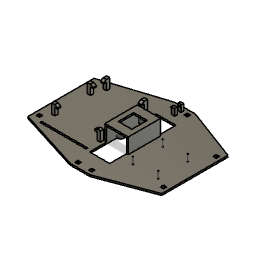
Seismo-Case v4 (Autodesk Fusion 360 design; units mm, degrees)
Autodesk Fusion 360 part; units mm, degrees
note: some values were not read from the file. Set by a fixed rule: which sketch regions a step uses.
sketch "Sketch1" plane through (0, 0, 0) normal (0, 1, 0) x (1, 0, 0)
  line L0 (-20, 30) -> (25.5, 30)
  line L1 (25.5, 30) -> (25.5, -33)
  line L2 (25.5, -33) -> (-20, -33)
  line L3 (-20, -33) -> (-20, 30)
  dimension "d1" = 63
  dimension "d2" = 45.5
  constraint horizontal L0
  constraint vertical L1
  constraint horizontal L2
  constraint vertical L3
  measures "d1" distance of L0.start L2.end
  measures "d2" distance of L0.start L0.end
extrude "Extrude1" add sketch "Sketch1" along normal blind 3.175 makes body 1
sketch "Sketch2" plane through (0, 0, 0) normal (0, -1, 0) x (1, 0, 0)
  line L0 (25.5, 33) -> (-20, 33)
  line L1 (-20, 33) -> (-20, -30)
  line L2 (-20, -30) -> (25.5, -30)
  line L3 (25.5, -30) -> (25.5, 33)
  circle A0 centre (2.225, 23.875) radius 6.2
  circle A1 centre (2.225, -20.875) radius 6.2
  dimension "d5" = 12.4
  dimension "d6" = 9.125
  dimension "d7" = 22.225
  dimension "d8" = 12.4
  dimension "d9" = 9.125
  dimension "d10" = 22.225
  measures "d5" diameter of A0
  measures "d6" distance of L0 A0.centre
  measures "d7" distance of L1 A0.centre
  measures "d8" diameter of A1
  measures "d9" distance of L2 A1.centre
  measures "d10" distance of L1 A1.centre
extrude "Extrude2" add sketch "Sketch2" along normal blind 12.065 contours A0 | A1 bodies 1
sketch "Sketch3" plane through (0, 0, 0) normal (0, -1, 0) x (1, 0, 0)
  circle A0 centre (2.225, -20.875) radius 6.2
  circle A1 centre (2.225, 23.875) radius 6.2
  line L0 (25.5, 33) -> (-20, 33)
  line L1 (-20, 33) -> (-20, -30)
  line L2 (-20, -30) -> (25.5, -30)
  line L3 (25.5, -30) -> (25.5, 33)
  line L4 (25.5, 33) -> (22.325, 33)
  line L5 (22.325, 33) -> (22.325, -30)
  line L6 (22.325, -30) -> (25.5, -30)
  line L7 (25.5, -30) -> (25.5, 33)
  line L8 (-20, 33) -> (-16.825, 33)
  line L9 (-16.825, 33) -> (-16.825, -30)
  line L10 (-16.825, -30) -> (-20, -30)
  line L11 (-20, -30) -> (-20, 33)
  dimension "d13" = 3.175
  dimension "d14" = 3.175
  constraint horizontal L4
  constraint vertical L5
  constraint horizontal L6
  constraint vertical L7
  constraint coincident L2 L5.end
  constraint coincident L0.start L3.end
  constraint horizontal L8
  constraint vertical L9
  constraint horizontal L10
  constraint vertical L11
  constraint coincident L0.end L1.start
  measures "d13" distance of L5 L7
  measures "d14" distance of L0.end L8.end
extrude "Extrude3" add sketch "Sketch3" along normal blind 26.67 contours L0 L2 L3 L4 L5 L6 L7 | L0 L1 L2 L8 L9 L10 L11 bodies 1
sketch "Sketch4" plane through (0, 3.175, 0) normal (0, 1, 0) x (-1, 0, 0)
  line L0 (20, 33) -> (-25.5, 33)
  line L1 (-25.5, 33) -> (-25.5, -30)
  line L2 (-25.5, -30) -> (20, -30)
  line L3 (20, -30) -> (20, 33)
  line L4 (10.475, -13.5) -> (-15.975, -13.5)
  line L5 (-15.975, -13.5) -> (-15.975, 16.5)
  line L6 (-15.975, 16.5) -> (10.475, 16.5)
  line L7 (10.475, 16.5) -> (10.475, -13.5)
  dimension "d17" = 16.5
  dimension "d18" = 16.5
  dimension "d19" = 9.525
  dimension "d20" = 9.525
  constraint horizontal L4
  constraint vertical L5
  constraint horizontal L6
  constraint vertical L7
  measures "d17" distance of L2 L4
  measures "d18" distance of L0 L6
  measures "d19" distance of L3 L7
  measures "d20" distance of L1 L5
extrude "Extrude4" cut sketch "Sketch4" against normal blind 22 contours L4 L5 L6 L7 bodies 1
ref_plane "WorkPlane1" through (23.9125, -26.67, 1.5) normal (0, -1, 0) x (0, 0, -1)
sketch "Sketch5" plane through (23.9125, -26.67, 1.5) normal (0, -1, 0) x (1, 0, 0)
  line L0 (-1.5875, -31.5) -> (-1.5875, -64.5)
  line L1 (-1.5875, 31.6383) -> (-1.5875, 64.6383)
  line L2 (-40.7375, 31.6383) -> (-40.7375, 64.6383)
  line L3 (-40.7375, -31.5) -> (-40.7375, -64.5)
  line L4 (-40.7375, -64.5) -> (-1.5875, -64.5)
  line L5 (-1.5875, 64.6383) -> (-40.7375, 64.6383)
  line L6 (-1.5875, -102.6) -> (100.0125, -64.5)
  line L7 (-1.5875, 102.7383) -> (100.0125, 64.6383)
  line L8 (-1.5875, -102.6) -> (-40.7375, -102.6)
  line L9 (-1.5875, 102.7383) -> (-40.7375, 102.7383)
  line L10 (-40.7375, 102.7383) -> (-160.7372, 64.9242)
  line L11 (100.0125, 64.6383) -> (100.0125, -64.5)
  line L12 (-1.5875, 31.6383) -> (-1.5875, 31.5)
  line L13 (-1.5875, 31.5) -> (1.6, 31.5)
  line L14 (1.6, 31.5) -> (1.6, -31.5)
  line L15 (-43.9125, -31.5) -> (-43.9125, 31.5)
  line L16 (-40.7375, 31.6383) -> (-40.7375, 31.5)
  line L17 (-40.7375, 31.5) -> (-43.9125, 31.5)
  line L18 (1.6, -31.5) -> (-1.5875, -31.5)
  line L19 (-40.7375, -31.5) -> (-43.9125, -31.5)
  line L20 (-160.7372, 64.9242) -> (-160.7372, -64.2138)
  line L21 (-40.7375, -102.6) -> (-160.7372, -64.2138)
  point P0 (-1.5875, -31.5)
  point P1 (-1.5875, 31.6383)
  point P2 (-43.9125, -31.5)
  point P3 (-43.9125, 31.5)
  point P4 (-40.7375, -31.5)
  point P5 (-40.7375, 31.6383)
  dimension "d28" = 33
  dimension "d29" = 33
  dimension "d30" = 33
  dimension "d31" = 33
  dimension "d32" = 38.1
  dimension "d35" = 101.6
  dimension "d37" = 38.1
  dimension "d38" = 120
  dimension "d40" = 38.1
  dimension "d41" = 38.1
  dimension "d42" = 129.1383
  dimension "d68" = 129.138
  constraint coincident P0 L0.start
  constraint coincident P1 L1.start
  constraint coincident P5 L2.start
  constraint vertical L2
  constraint coincident P4 L3.start
  constraint vertical L3
  constraint perpendicular L0 L4
  constraint perpendicular L1 L5
  constraint parallel L1 L12
  constraint perpendicular L13 L14
  constraint coincident P2 L15.start
  constraint coincident P3 L15.end
  constraint parallel L3 L15
  constraint parallel L15 L16
  constraint perpendicular L15 L17
  constraint perpendicular L15 L19
  constraint vertical L20
  measures "d28" distance of P0 L0.end
  measures "d29" distance of P1 L1.end
  measures "d30" distance of P5 L2.end
  measures "d31" distance of P4 L3.end
  measures "d32" distance of L0.end L6.start
  measures "d35" distance of L0.end L6.end
  measures "d37" distance of L1.end L7.start
  measures "d38" distance of L2.end L10.end
  measures "d40" distance of L3.end L8.end
  measures "d41" distance of L2.end L9.end
  measures "d42" distance of L6.end L7.end
  measures "d68" distance of L10.end L20.end
extrude "Extrude5" add sketch "Sketch5" along normal blind 3.175 separate body makes body 2
sketch "Sketch6" plane through (0, -26.67, 0) normal (0, 1, 0) x (-1, 0, 0)
  line L0 (16.825, -63) -> (-22.325, -63)
  line L1 (-22.325, -63) -> (-22.325, -30)
  line L2 (-22.325, -30) -> (-25.5125, -30)
  line L3 (-25.5125, -30) -> (-25.5125, 33)
  line L4 (-25.5125, 33) -> (-22.325, 33)
  line L5 (-22.325, 33) -> (-22.325, 66.1383)
  line L6 (-22.325, 66.1383) -> (16.825, 66.1383)
  line L7 (16.825, 66.1383) -> (16.825, 33)
  line L8 (16.825, 33) -> (20, 33)
  line L9 (20, 33) -> (20, -30)
  line L10 (20, -30) -> (16.825, -30)
  line L11 (16.825, -30) -> (16.825, -63)
  line L12 (16.825, 104.2383) -> (-22.325, 104.2383)
  line L13 (-22.325, 104.2383) -> (-123.925, 66.1383)
  line L14 (-123.925, 66.1383) -> (-123.925, -63)
  line L15 (-123.925, -63) -> (-22.325, -101.1)
  line L16 (-22.325, -101.1) -> (16.825, -101.1)
  line L17 (136.8247, 66.4242) -> (16.825, 104.2383)
  line L18 (0.425, -95) -> (-5.925, -95)
  line L19 (-5.925, -95) -> (-5.925, -89.92)
  line L20 (-5.925, -89.92) -> (0.425, -89.92)
  line L21 (0.425, -89.92) -> (0.425, -95)
  line L22 (0.425, -82.3) -> (-5.925, -82.3)
  line L23 (-5.925, -82.3) -> (-5.925, -77.22)
  line L24 (-5.925, -77.22) -> (0.425, -77.22)
  line L25 (0.425, -77.22) -> (0.425, -82.3)
  line L26 (16.825, -101.1) -> (136.8247, -62.7138)
  line L27 (136.8247, -62.7138) -> (136.8247, 66.4242)
  dimension "d45" = 6.35
  dimension "d46" = 5.08
  dimension "d48" = 16.4
  dimension "d50" = 6.35
  dimension "d51" = 5.08
  dimension "d52" = 16.4
  dimension "d53" = 7.62
  constraint horizontal L18
  constraint vertical L19
  constraint horizontal L20
  constraint vertical L21
  constraint horizontal L22
  constraint vertical L23
  constraint horizontal L24
  constraint vertical L25
  measures "d45" distance of L18.start L18.end
  measures "d46" distance of L18.end L19.end
  measures "d48" distance of L11 L21
  measures "d50" distance of L22.start L22.end
  measures "d51" distance of L22.end L23.end
  measures "d52" distance of L11 L25
  measures "d53" distance of L20 L22
extrude "Extrude6" add sketch "Sketch6" along normal blind 12.7 contours L18 L19 L20 L21 | L22 L23 L24 L25 bodies 2
sketch "Sketch7" plane through (5.925, 0, 0) normal (1, 0, 0) x (0, 0, -1)
  line L0 (77.22, -26.67) -> (82.3, -26.67)
  line L1 (82.3, -26.67) -> (82.3, -13.97)
  line L2 (82.3, -13.97) -> (77.22, -13.97)
  line L3 (77.22, -13.97) -> (77.22, -26.67)
  line L4 (83.57, -16) -> (83.57, -17)
  line L5 (88.65, -16) -> (88.65, -17)
  line L6 (83.57, -16) -> (82.3, -13.97)
  line L7 (83.57, -17) -> (82.3, -17)
  line L8 (88.65, -17) -> (89.92, -17)
  line L9 (89.92, -13.97) -> (88.65, -16)
  line L10 (89.92, -13.97) -> (89.92, -17)
  point P0 (89.92, -13.97)
  dimension "d56" = 5.08
  dimension "d58" = 1.27
  constraint perpendicular L2 L4
  constraint vertical L5
  constraint coincident L1.end L2.start
  constraint coincident L1 L7.end
  constraint perpendicular L1 L7
  constraint perpendicular L5 L8
  constraint coincident P0 L9.start
  constraint perpendicular L8 L10
  measures "d56" distance of L4.start L5.start
  measures "d58" distance of L1 L4.start
extrude "Extrude7" add sketch "Sketch7" against normal blind 6.35 contours L1 L4 L6 L7 | L5 L8 L9 L10 bodies 2
sketch "Sketch8" plane through (0, -26.67, 0) normal (0, 1, 0) x (-1, 0, 0)
  line L0 (0.425, -77.22) -> (0.425, -82.3)
  line L1 (0.425, -82.3) -> (-5.925, -82.3)
  line L2 (-5.925, -82.3) -> (-5.925, -77.22)
  line L3 (-5.925, -77.22) -> (0.425, -77.22)
  line L4 (0.425, -89.92) -> (0.425, -95)
  line L5 (0.425, -95) -> (-5.925, -95)
  line L6 (-5.925, -95) -> (-5.925, -89.92)
  line L7 (-5.925, -89.92) -> (0.425, -89.92)
  line L8 (16.825, -63) -> (-22.325, -63)
  line L9 (-22.325, -63) -> (-22.325, -30)
  line L10 (-22.325, -30) -> (-25.5125, -30)
  line L11 (-25.5125, -30) -> (-25.5125, 33)
  line L12 (-25.5125, 33) -> (-22.325, 33)
  line L13 (-22.325, 33) -> (-22.325, 66.1383)
  line L14 (-22.325, 66.1383) -> (16.825, 66.1383)
  line L15 (16.825, 66.1383) -> (16.825, 33)
  line L16 (16.825, 33) -> (20, 33)
  line L17 (20, 33) -> (20, -30)
  line L18 (20, -30) -> (16.825, -30)
  line L19 (16.825, -30) -> (16.825, -63)
  line L20 (16.825, 104.2383) -> (-22.325, 104.2383)
  line L21 (-22.325, 104.2383) -> (-123.925, 66.1383)
  line L22 (-123.925, 66.1383) -> (-123.925, -63)
  line L23 (-123.925, -63) -> (-22.325, -101.1)
  line L24 (-22.325, -101.1) -> (16.825, -101.1)
  line L25 (136.8247, 66.4242) -> (16.825, 104.2383)
  line L26 (111.4247, -51.1) -> (28.8747, -51.1)
  line L27 (28.8747, -51.1) -> (28.8747, 65.105)
  line L28 (28.8747, 65.105) -> (111.4247, 65.105)
  line L29 (111.4247, 65.105) -> (111.4247, -51.1)
  line L30 (16.825, -101.1) -> (136.8247, -62.7138)
  line L31 (136.8247, -62.7138) -> (136.8247, 66.4242)
  line L32 (59.9342, -51.1) -> (59.9342, -70.15)
  line L33 (114.5997, 68.28) -> (25.6997, 68.28)
  line L34 (25.6997, 68.28) -> (25.6997, 65.105)
  line L35 (25.6997, 65.105) -> (28.8747, 65.105)
  line L36 (114.5997, 68.28) -> (114.5997, 65.105)
  line L37 (114.5997, 65.105) -> (111.4247, 65.105)
  line L38 (-34.3875, -41.7617) -> (-94.3875, -41.7617)
  line L39 (-94.3875, -41.7617) -> (-94.3875, 47.2383)
  line L40 (-94.3875, 47.2383) -> (-34.3875, 47.2383)
  line L41 (-34.3875, 47.2383) -> (-34.3875, -41.7617)
  line L42 (28.8747, 33) -> (22.5247, 33)
  line L43 (22.5247, 33) -> (22.5247, 39.35)
  line L44 (22.5247, 39.35) -> (28.8747, 39.35)
  line L45 (28.8747, 39.35) -> (28.8747, 33)
  line L46 (111.4247, 33) -> (117.7747, 33)
  line L47 (117.7747, 33) -> (117.7747, 39.35)
  line L48 (117.7747, 39.35) -> (111.4247, 39.35)
  line L49 (111.4247, 39.35) -> (111.4247, 33)
  line L50 (28.8747, -30.0326) -> (22.5247, -30.0326)
  line L51 (22.5247, -30.0326) -> (22.5247, -36.3826)
  line L52 (22.5247, -36.3826) -> (28.8747, -36.3826)
  line L53 (28.8747, -36.3826) -> (28.8747, -30.0326)
  line L54 (111.4247, -36.3826) -> (117.7747, -36.3826)
  line L55 (117.7747, -36.3826) -> (117.7747, -30.0326)
  line L56 (117.7747, -30.0326) -> (111.4247, -30.0326)
  line L57 (111.4247, -30.0326) -> (111.4247, -36.3826)
  dimension "d61" = 82.55
  dimension "d62" = 116.205
  dimension "d64" = 50
  dimension "d65" = 39.1333
  dimension "d69" = 25.4
  dimension "d70" = 19.05
  dimension "d71" = 3.175
  dimension "d72" = 3.175
  dimension "d73" = 3.175
  dimension "d74" = 89
  dimension "d75" = 60
  dimension "d78" = 57
  dimension "d79" = 59.3383
  dimension "d80" = 6.35
  dimension "d81" = 6.35
  dimension "d82" = 8.8747
  dimension "d83" = 8.875
  dimension "d84" = 6.35
  dimension "d85" = 6.35
  dimension "d86" = 6.35
  dimension "d87" = 6.35
  dimension "d88" = 6.35
  dimension "d89" = 6.35
  constraint horizontal L26
  constraint vertical L27
  constraint horizontal L28
  constraint vertical L29
  constraint coincident L26 L32.start
  constraint perpendicular L26 L32
  constraint perpendicular L29 L33
  constraint perpendicular L33 L34
  constraint perpendicular L27 L35
  constraint perpendicular L33 L36
  constraint perpendicular L36 L37
  constraint horizontal L38
  constraint vertical L39
  constraint horizontal L40
  constraint vertical L41
  constraint horizontal L42
  constraint vertical L43
  constraint horizontal L44
  constraint vertical L45
  constraint coincident L27 L42.start
  constraint horizontal L46
  constraint vertical L47
  constraint horizontal L48
  constraint vertical L49
  constraint coincident L29 L46.start
  constraint horizontal L50
  constraint vertical L51
  constraint horizontal L52
  constraint vertical L53
  constraint coincident L27 L50.start
  constraint horizontal L54
  constraint vertical L55
  constraint horizontal L56
  constraint vertical L57
  constraint coincident L29 L54.start
  measures "d61" distance of L26.start L26.end
  measures "d62" distance of L26.start L28.end
  measures "d64" distance of L24 L26
  measures "d65" distance of L20 L28
  measures "d69" distance of L29 L31
  measures "d70" distance of L32.start L32.end
  measures "d71" distance of L28 L33
  measures "d72" distance of L29 L36
  measures "d73" distance of L27 L34
  measures "d74" distance of L38.end L39.end
  measures "d75" distance of L39.end L40.end
  measures "d78" distance of L20 L40
  measures "d79" distance of L24 L38
  measures "d80" distance of L42.start L42.end
  measures "d81" distance of L42 L44
  measures "d82" distance of L17 L27
  measures "d83" distance of L11 L41
  measures "d84" distance of L46.start L46.end
  measures "d85" distance of L46 L48
  measures "d86" distance of L50.start L50.end
  measures "d87" distance of L50 L52
  measures "d88" distance of L54.start L54.end
  measures "d89" distance of L54 L56
extrude "Extrude8" add sketch "Sketch8" along normal blind 19.05 contours L29 L54 L55 L56 L57 | L27 L50 L51 L52 L53 | L29 L46 L47 L48 L49 | L27 L42 L43 L44 L45 bodies 2
sketch "Sketch9" plane through (0, 0, 39.35) normal (0, 0, 1) x (1, 0, 0)
  line L0 (-117.7747, -26.67) -> (-111.4247, -26.67)
  line L1 (-111.4247, -26.67) -> (-111.4247, -7.62)
  line L2 (-111.4247, -7.62) -> (-117.7747, -7.62)
  line L3 (-117.7747, -7.62) -> (-117.7747, -26.67)
  line L4 (-111.4247, -7.62) -> (-105.9254, -10.795)
  line L5 (-105.9254, -10.795) -> (-105.9254, -12.3825)
  line L6 (-105.9254, -12.3825) -> (-111.4247, -12.3825)
  line L7 (-111.4247, -7.62) -> (-111.4247, -12.3825)
  line L8 (-34.3739, -10.795) -> (-34.3739, -12.383)
  line L9 (-28.8747, -7.62) -> (-34.3739, -10.795)
  line L10 (-28.8747, -7.62) -> (-28.8747, -12.383)
  line L11 (-28.8747, -12.383) -> (-34.3739, -12.383)
  point P0 (-28.8747, -7.62)
  dimension "d92" = 6.35
  dimension "d93" = 120
  dimension "d94" = 1.5875
  dimension "d98" = 1.588
  dimension "d101" = 6.35
  dimension "d102" = 90
  dimension "d103" = 120
  constraint coincident L1.end L2.start
  constraint vertical L5
  constraint coincident L1 L6.end
  constraint perpendicular L1 L6
  constraint vertical L8
  constraint coincident P0 L9.start
  constraint vertical L10
  measures "d92" distance of L1.end L4.end
  measures "d93" angle of L1 L4
  measures "d94" distance of L4.end L5.end
  measures "d98" distance of L8.start L8.end
  measures "d101" distance of L8.start P0
  measures "d102" angle of L10 L11
  measures "d103" angle of L9 L10
extrude "Extrude9" add sketch "Sketch9" against normal blind 6.35 contours L1 L4 L5 L6 L7 | L8 L9 L10 L11 bodies 2
sketch "Sketch10" plane through (0, 0, -36.3826) normal (0, 0, -1) x (-1, 0, 0)
  line L0 (22.5247, -26.67) -> (28.8747, -26.67)
  line L1 (28.8747, -26.67) -> (28.8747, -7.62)
  line L2 (28.8747, -7.62) -> (22.5247, -7.62)
  line L3 (22.5247, -7.62) -> (22.5247, -26.67)
  line L4 (28.8747, -7.62) -> (34.3739, -10.795)
  line L5 (34.3739, -10.795) -> (34.3739, -12.3825)
  line L6 (34.3739, -12.3825) -> (28.8747, -12.3825)
  line L7 (28.8747, -7.62) -> (28.8747, -12.3825)
  dimension "d107" = 6.35
  dimension "d108" = 120
  dimension "d109" = 1.5875
  constraint coincident L1.end L2.start
  constraint parallel L1 L5
  constraint coincident L1 L6.end
  constraint perpendicular L1 L6
  constraint perpendicular L6 L7
  measures "d107" distance of L1.end L4.end
  measures "d108" angle of L4 L7
  measures "d109" distance of L4.end L5.end
extrude "Extrude10" add sketch "Sketch10" against normal blind 6.35 contours L1 L4 L5 L6 L7 bodies 2
sketch "Sketch11" plane through (0, 0, -30.0326) normal (0, 0, 1) x (1, 0, 0)
  line L0 (-117.7747, -26.67) -> (-111.4247, -26.67)
  line L1 (-111.4247, -26.67) -> (-111.4247, -7.62)
  line L2 (-111.4247, -7.62) -> (-117.7747, -7.62)
  line L3 (-117.7747, -7.62) -> (-117.7747, -26.67)
  line L4 (-111.4247, -7.62) -> (-105.9212, -10.7878)
  line L5 (-105.9212, -10.7878) -> (-105.9212, -12.4)
  line L6 (-105.9212, -12.4) -> (-111.4247, -12.4)
  line L7 (-111.4247, -7.62) -> (-111.4247, -12.4)
  dimension "d113" = 6.35
  constraint coincident L1.end L2.start
  constraint vertical L5
  constraint coincident L1 L6.end
  constraint perpendicular L1 L6
  measures "d113" distance of L1.end L4.end
extrude "Extrude11" add sketch "Sketch11" against normal blind 6.35 contours L1 L4 L5 L6 L7 bodies 2
sketch "Sketch12" plane through (0, -29.845, 0) normal (0, -1, 0) x (1, 0, 0)
  line L0 (22.325, -63) -> (-16.825, -63)
  line L1 (-16.825, -63) -> (-16.825, -30)
  line L2 (-16.825, -30) -> (-20, -30)
  line L3 (-20, -30) -> (-20, 33)
  line L4 (-20, 33) -> (-16.825, 33)
  line L5 (-16.825, 33) -> (-16.825, 66.1383)
  line L6 (-16.825, 66.1383) -> (22.325, 66.1383)
  line L7 (22.325, 66.1383) -> (22.325, 33)
  line L8 (22.325, 33) -> (25.5125, 33)
  line L9 (25.5125, 33) -> (25.5125, -30)
  line L10 (25.5125, -30) -> (22.325, -30)
  line L11 (22.325, -30) -> (22.325, -63)
  line L12 (22.325, -101.1) -> (123.925, -63)
  line L13 (123.925, -63) -> (123.925, 66.1383)
  line L14 (123.925, 66.1383) -> (22.325, 104.2383)
  line L15 (22.325, 104.2383) -> (-16.825, 104.2383)
  line L16 (-16.825, 104.2383) -> (-136.8247, 66.4242)
  line L17 (-136.8247, 66.4242) -> (-136.8247, -62.7138)
  line L18 (-136.8247, -62.7138) -> (-16.825, -101.1)
  line L19 (-16.825, -101.1) -> (22.325, -101.1)
  line L20 (-16.825, 33) -> (-20, 33)
  line L21 (-20, 33) -> (-20, -30)
  line L22 (-20, -30) -> (-16.825, -30)
  line L23 (-16.825, -30) -> (-16.825, 33)
  line L24 (22.325, 33) -> (25.5125, 33)
  line L25 (25.5125, 33) -> (25.5125, -30)
  line L26 (25.5125, -30) -> (22.325, -30)
  line L27 (22.325, -30) -> (22.325, 33)
  constraint horizontal L20
  constraint vertical L21
  constraint horizontal L22
  constraint vertical L23
  constraint coincident L2.end L3.start
  constraint coincident L4.end L5.start
  constraint horizontal L24
  constraint vertical L25
  constraint horizontal L26
  constraint vertical L27
  constraint coincident L9.end L10.start
  constraint coincident L7.end L8.start
extrude "Extrude12" add sketch "Sketch12" against normal blind 3.175 contours L8 L9 L10 L24 L25 L26 L27 | L2 L3 L4 L20 L21 L22 L23 bodies 1 2
sketch "Sketch13" plane through (0, -26.67, 0) normal (0, 1, 0) x (-1, 0, 0)
  line L0 (111.4247, 39.35) -> (117.7747, 39.35)
  line L1 (117.7747, 39.35) -> (117.7747, 33)
  line L2 (117.7747, 33) -> (111.4247, 33)
  line L3 (111.4247, 33) -> (111.4247, 39.35)
  line L4 (111.4247, -30.0326) -> (117.7747, -30.0326)
  line L5 (117.7747, -30.0326) -> (117.7747, -36.3826)
  line L6 (117.7747, -36.3826) -> (111.4247, -36.3826)
  line L7 (111.4247, -36.3826) -> (111.4247, -30.0326)
  line L8 (28.8747, 39.35) -> (28.8747, 33)
  line L9 (28.8747, 33) -> (22.5247, 33)
  line L10 (22.5247, 33) -> (22.5247, 39.35)
  line L11 (22.5247, 39.35) -> (28.8747, 39.35)
  line L12 (28.8747, -36.3826) -> (22.5247, -36.3826)
  line L13 (22.5247, -36.3826) -> (22.5247, -30.0326)
  line L14 (22.5247, -30.0326) -> (28.8747, -30.0326)
  line L15 (28.8747, -30.0326) -> (28.8747, -36.3826)
  line L16 (0.425, -77.22) -> (0.425, -82.3)
  line L17 (0.425, -82.3) -> (-5.925, -82.3)
  line L18 (-5.925, -82.3) -> (-5.925, -77.22)
  line L19 (-5.925, -77.22) -> (0.425, -77.22)
  line L20 (0.425, -89.92) -> (0.425, -95)
  line L21 (0.425, -95) -> (-5.925, -95)
  line L22 (-5.925, -95) -> (-5.925, -89.92)
  line L23 (-5.925, -89.92) -> (0.425, -89.92)
  line L24 (16.825, -63) -> (-22.325, -63)
  line L25 (-22.325, -63) -> (-22.325, -30)
  line L26 (-22.325, -30) -> (-25.5, -30)
  line L27 (-25.5, -30) -> (-25.5, 33)
  line L28 (-25.5, 33) -> (-22.325, 33)
  line L29 (-22.325, 33) -> (-22.325, -30)
  line L30 (-22.325, -30) -> (-22.325, -30)
  line L31 (-22.325, -30) -> (-22.325, 66.1383)
  line L32 (-22.325, 66.1383) -> (16.825, 66.1383)
  line L33 (16.825, 66.1383) -> (16.825, 33)
  line L34 (16.825, 33) -> (20, 33)
  line L35 (20, 33) -> (20, -30)
  line L36 (20, -30) -> (16.825, -30)
  line L37 (16.825, -30) -> (16.825, -63)
  line L38 (-123.925, -63) -> (-22.325, -101.1)
  line L39 (-22.325, -101.1) -> (16.825, -101.1)
  line L40 (16.825, -101.1) -> (136.8247, -62.7138)
  line L41 (136.8247, -62.7138) -> (136.8247, 66.4242)
  line L42 (136.8247, 66.4242) -> (16.825, 104.2383)
  line L43 (16.825, 104.2383) -> (-22.325, 104.2383)
  line L44 (-22.325, 104.2383) -> (-123.925, 66.1383)
  line L45 (-123.925, 66.1383) -> (-123.925, -63)
  line L46 (110, -60) -> (103.65, -60)
  line L47 (103.65, -60) -> (103.65, -53.65)
  line L48 (103.65, -53.65) -> (110, -53.65)
  line L49 (110, -53.65) -> (110, -60)
  line L50 (30, -60) -> (36.35, -60)
  line L51 (36.35, -60) -> (36.35, -53.65)
  line L52 (36.35, -53.65) -> (30, -53.65)
  line L53 (30, -53.65) -> (30, -60)
  line L54 (111.4247, 64.46) -> (28.0914, 64.46)
  dimension "d118" = 6.35
  dimension "d119" = 6.35
  dimension "d120" = 6.35
  dimension "d121" = 6.35
  dimension "d122" = 118.11
  constraint horizontal L46
  constraint vertical L47
  constraint horizontal L48
  constraint vertical L49
  constraint horizontal L50
  constraint vertical L51
  constraint horizontal L52
  constraint vertical L53
  constraint perpendicular L3 L54
  measures "d118" distance of L46.start L46.end
  measures "d119" distance of L46.start L48.end
  measures "d120" distance of L50.start L50.end
  measures "d121" distance of L50.end L51.end
  measures "d122" distance of L48 L54
extrude "Extrude13" add sketch "Sketch13" along normal blind 19.05 contours L46 L47 L48 L49 | L50 L51 L52 L53 bodies 1
sketch "Sketch14" plane through (-110, 0, 0) normal (-1, 0, 0) x (0, 0, 1)
  line L0 (-60, -26.67) -> (-53.65, -26.67)
  line L1 (-53.65, -26.67) -> (-53.65, -7.62)
  line L2 (-53.65, -7.62) -> (-60, -7.62)
  line L3 (-60, -7.62) -> (-60, -26.67)
  line L4 (-48.15, -10.7937) -> (-48.15, -12.3817)
  line L5 (-48.15, -10.7937) -> (-53.65, -7.62)
  line L6 (-48.15, -12.3817) -> (-53.65, -12.3817)
  dimension "d125" = 1.588
  dimension "d126" = 5.5
  dimension "d127" = 6.35
  constraint vertical L4
  constraint coincident L1.end L2.start
  constraint coincident L1 L6.end
  constraint perpendicular L1 L6
  measures "d125" distance of L4.start L4.end
  measures "d126" distance of L1 L4
  measures "d127" distance of L4.start L1.end
extrude "Extrude14" add sketch "Sketch14" against normal blind 6.35 contours L1 L4 L5 L6 bodies 1
sketch "Sketch15" plane through (-30, 0, 0) normal (1, 0, 0) x (0, 0, -1)
  line L0 (53.65, -26.67) -> (60, -26.67)
  line L1 (60, -26.67) -> (60, -7.62)
  line L2 (60, -7.62) -> (53.65, -7.62)
  line L3 (53.65, -7.62) -> (53.65, -26.67)
  line L4 (48.15, -12.3946) -> (48.15, -10.8066)
  line L5 (48.15, -12.3946) -> (53.65, -12.3946)
  line L6 (53.65, -7.62) -> (53.65, -12.3946)
  line L7 (53.65, -7.62) -> (48.15, -10.8066)
  dimension "d130" = 1.588
  dimension "d131" = 5.5
  constraint vertical L4
  constraint coincident L3 L5.end
  constraint perpendicular L3 L5
  constraint coincident L2.end L3.start
  constraint perpendicular L5 L6
  measures "d130" distance of L4.start L4.end
  measures "d131" distance of L3 L4
extrude "Extrude15" add sketch "Sketch15" against normal blind 6.35 contours L3 L4 L5 L6 L7 bodies 1
sketch "Sketch16" plane through (0, -26.67, 0) normal (0, 1, 0) x (-1, 0, 0)
  line L0 (30, -53.65) -> (36.35, -53.65)
  line L1 (36.35, -53.65) -> (36.35, -60)
  line L2 (36.35, -60) -> (30, -60)
  line L3 (30, -60) -> (30, -53.65)
  line L4 (110, -53.65) -> (110, -60)
  line L5 (110, -60) -> (103.65, -60)
  line L6 (103.65, -60) -> (103.65, -53.65)
  line L7 (103.65, -53.65) -> (110, -53.65)
  line L8 (111.4247, 39.35) -> (117.7747, 39.35)
  line L9 (117.7747, 39.35) -> (117.7747, 33)
  line L10 (117.7747, 33) -> (111.4247, 33)
  line L11 (111.4247, 33) -> (111.4247, 39.35)
  line L12 (111.4247, -30.0326) -> (117.7747, -30.0326)
  line L13 (117.7747, -30.0326) -> (117.7747, -36.3826)
  line L14 (117.7747, -36.3826) -> (111.4247, -36.3826)
  line L15 (111.4247, -36.3826) -> (111.4247, -30.0326)
  line L16 (28.8747, 39.35) -> (28.8747, 33)
  line L17 (28.8747, 33) -> (22.5247, 33)
  line L18 (22.5247, 33) -> (22.5247, 39.35)
  line L19 (22.5247, 39.35) -> (28.8747, 39.35)
  line L20 (28.8747, -36.3826) -> (22.5247, -36.3826)
  line L21 (22.5247, -36.3826) -> (22.5247, -30.0326)
  line L22 (22.5247, -30.0326) -> (28.8747, -30.0326)
  line L23 (28.8747, -30.0326) -> (28.8747, -36.3826)
  line L24 (0.425, -77.22) -> (0.425, -82.3)
  line L25 (0.425, -82.3) -> (-5.925, -82.3)
  line L26 (-5.925, -82.3) -> (-5.925, -77.22)
  line L27 (-5.925, -77.22) -> (0.425, -77.22)
  line L28 (0.425, -89.92) -> (0.425, -95)
  line L29 (0.425, -95) -> (-5.925, -95)
  line L30 (-5.925, -95) -> (-5.925, -89.92)
  line L31 (-5.925, -89.92) -> (0.425, -89.92)
  line L32 (16.825, -63) -> (-22.325, -63)
  line L33 (-22.325, -63) -> (-22.325, -30)
  line L34 (-22.325, -30) -> (-25.5, -30)
  line L35 (-25.5, -30) -> (-25.5, 33)
  line L36 (-25.5, 33) -> (-22.325, 33)
  line L37 (-22.325, 33) -> (-22.325, -30)
  line L38 (-22.325, -30) -> (-22.325, -30)
  line L39 (-22.325, -30) -> (-22.325, 66.1383)
  line L40 (-22.325, 66.1383) -> (16.825, 66.1383)
  line L41 (16.825, 66.1383) -> (16.825, 33)
  line L42 (16.825, 33) -> (20, 33)
  line L43 (20, 33) -> (20, -30)
  line L44 (20, -30) -> (16.825, -30)
  line L45 (16.825, -30) -> (16.825, -63)
  line L46 (-123.925, -63) -> (-22.325, -101.1)
  line L47 (-22.325, -101.1) -> (16.825, -101.1)
  line L48 (16.825, -101.1) -> (136.8247, -62.7138)
  line L49 (136.8247, -62.7138) -> (136.8247, 66.4242)
  line L50 (136.8247, 66.4242) -> (16.825, 104.2383)
  line L51 (16.825, 104.2383) -> (-22.325, 104.2383)
  line L52 (-22.325, 104.2383) -> (-123.925, 66.1383)
  line L53 (-123.925, 66.1383) -> (-123.925, -63)
  line L54 (115.2747, 61.35) -> (25.2747, 61.35)
  line L55 (115.2747, 61.35) -> (115.2747, 64.6012)
  line L56 (115.2747, 64.6012) -> (25.2747, 64.6012)
  line L57 (25.2747, 64.6012) -> (25.2747, 61.35)
  dimension "d135" = 90
  dimension "d136" = 2.5
  dimension "d137" = 3.2512
  dimension "d138" = 90
  constraint horizontal L54
  constraint perpendicular L54 L55
  constraint perpendicular L49 L56
  measures "d135" distance of L54.start L54.end
  measures "d136" horizontal distance of L8.end L54.start
  measures "d137" distance of L54.start L55.end
  measures "d138" distance of L55.end L56.end
extrude "Extrude16" cut sketch "Sketch16" against normal blind 100 contours L54 L55 L56 L57 bodies 1
sketch "Sketch17" plane through (0, -26.67, 0) normal (0, 1, 0) x (-1, 0, 0)
  line L0 (25.2747, 64.6012) -> (115.2747, 64.6012)
  line L1 (115.2747, 64.6012) -> (115.2747, 61.35)
  line L2 (115.2747, 61.35) -> (25.2747, 61.35)
  line L3 (25.2747, 61.35) -> (25.2747, 64.6012)
  line L4 (30, -53.65) -> (36.35, -53.65)
  line L5 (36.35, -53.65) -> (36.35, -60)
  line L6 (36.35, -60) -> (30, -60)
  line L7 (30, -60) -> (30, -53.65)
  line L8 (110, -53.65) -> (110, -60)
  line L9 (110, -60) -> (103.65, -60)
  line L10 (103.65, -60) -> (103.65, -53.65)
  line L11 (103.65, -53.65) -> (110, -53.65)
  line L12 (111.4247, 39.35) -> (117.7747, 39.35)
  line L13 (117.7747, 39.35) -> (117.7747, 33)
  line L14 (117.7747, 33) -> (111.4247, 33)
  line L15 (111.4247, 33) -> (111.4247, 39.35)
  line L16 (111.4247, -30.0326) -> (117.7747, -30.0326)
  line L17 (117.7747, -30.0326) -> (117.7747, -36.3826)
  line L18 (117.7747, -36.3826) -> (111.4247, -36.3826)
  line L19 (111.4247, -36.3826) -> (111.4247, -30.0326)
  line L20 (28.8747, 39.35) -> (28.8747, 33)
  line L21 (28.8747, 33) -> (22.5247, 33)
  line L22 (22.5247, 33) -> (22.5247, 39.35)
  line L23 (22.5247, 39.35) -> (28.8747, 39.35)
  line L24 (28.8747, -36.3826) -> (22.5247, -36.3826)
  line L25 (22.5247, -36.3826) -> (22.5247, -30.0326)
  line L26 (22.5247, -30.0326) -> (28.8747, -30.0326)
  line L27 (28.8747, -30.0326) -> (28.8747, -36.3826)
  line L28 (0.425, -77.22) -> (0.425, -82.3)
  line L29 (0.425, -82.3) -> (-5.925, -82.3)
  line L30 (-5.925, -82.3) -> (-5.925, -77.22)
  line L31 (-5.925, -77.22) -> (0.425, -77.22)
  line L32 (0.425, -89.92) -> (0.425, -95)
  line L33 (0.425, -95) -> (-5.925, -95)
  line L34 (-5.925, -95) -> (-5.925, -89.92)
  line L35 (-5.925, -89.92) -> (0.425, -89.92)
  line L36 (16.825, -63) -> (-22.325, -63)
  line L37 (-22.325, -63) -> (-22.325, -30)
  line L38 (-22.325, -30) -> (-25.5, -30)
  line L39 (-25.5, -30) -> (-25.5, 33)
  line L40 (-25.5, 33) -> (-22.325, 33)
  line L41 (-22.325, 33) -> (-22.325, -30)
  line L42 (-22.325, -30) -> (-22.325, -30)
  line L43 (-22.325, -30) -> (-22.325, 66.1383)
  line L44 (-22.325, 66.1383) -> (16.825, 66.1383)
  line L45 (16.825, 66.1383) -> (16.825, 33)
  line L46 (16.825, 33) -> (20, 33)
  line L47 (20, 33) -> (20, -30)
  line L48 (20, -30) -> (16.825, -30)
  line L49 (16.825, -30) -> (16.825, -63)
  line L50 (-123.925, -63) -> (-22.325, -101.1)
  line L51 (-22.325, -101.1) -> (16.825, -101.1)
  line L52 (16.825, -101.1) -> (136.8247, -62.7138)
  line L53 (136.8247, -62.7138) -> (136.8247, 66.4242)
  line L54 (136.8247, 66.4242) -> (16.825, 104.2383)
  line L55 (16.825, 104.2383) -> (-22.325, 104.2383)
  line L56 (-22.325, 104.2383) -> (-123.925, 66.1383)
  line L57 (-123.925, 66.1383) -> (-123.925, -63)
  circle A0 centre (-95, -13.7617) radius 1.275
  circle A1 centre (-95, 44.2383) radius 1.275
  circle A2 centre (-46, 44.2383) radius 1.275
  circle A3 centre (-46, -13.7617) radius 1.275
  dimension "d155" = 2.55
  dimension "d156" = 2.55
  dimension "d157" = 2.55
  dimension "d158" = 2.55
  dimension "d159" = 58
  dimension "d161" = 49
  dimension "d163" = 60
  dimension "d164" = 60
  dimension "d165" = 58
  dimension "d166" = 49
  measures "d155" diameter of A0
  measures "d156" diameter of A1
  measures "d157" diameter of A2
  measures "d158" diameter of A3
  measures "d159" distance of A2.centre A3.centre
  measures "d161" horizontal distance of A0.centre A3.centre
  measures "d163" distance of L55 A2.centre
  measures "d164" distance of L55 A1.centre
  measures "d165" vertical distance of A0.centre A1.centre
  measures "d166" distance of A1.centre A2.centre
extrude "Extrude17" add sketch "Sketch17" along normal blind 12.7 contours A0 | A1 | A2 | A3 bodies 1
sketch "Sketch18" plane through (0, -26.67, 0) normal (0, 1, 0) x (-1, 0, 0)
  circle A0 centre (-95, -13.7617) radius 1.275
  circle A1 centre (-46, 44.2383) radius 1.275
  circle A2 centre (-95, 44.2383) radius 1.275
  circle A3 centre (-46, -13.7617) radius 1.275
  line L0 (25.2747, 64.6012) -> (115.2747, 64.6012)
  line L1 (115.2747, 64.6012) -> (115.2747, 61.35)
  line L2 (115.2747, 61.35) -> (25.2747, 61.35)
  line L3 (25.2747, 61.35) -> (25.2747, 64.6012)
  line L4 (30, -53.65) -> (36.35, -53.65)
  line L5 (36.35, -53.65) -> (36.35, -60)
  line L6 (36.35, -60) -> (30, -60)
  line L7 (30, -60) -> (30, -53.65)
  line L8 (110, -53.65) -> (110, -60)
  line L9 (110, -60) -> (103.65, -60)
  line L10 (103.65, -60) -> (103.65, -53.65)
  line L11 (103.65, -53.65) -> (110, -53.65)
  line L12 (111.4247, 39.35) -> (117.7747, 39.35)
  line L13 (117.7747, 39.35) -> (117.7747, 33)
  line L14 (117.7747, 33) -> (111.4247, 33)
  line L15 (111.4247, 33) -> (111.4247, 39.35)
  line L16 (111.4247, -30.0326) -> (117.7747, -30.0326)
  line L17 (117.7747, -30.0326) -> (117.7747, -36.3826)
  line L18 (117.7747, -36.3826) -> (111.4247, -36.3826)
  line L19 (111.4247, -36.3826) -> (111.4247, -30.0326)
  line L20 (28.8747, 39.35) -> (28.8747, 33)
  line L21 (28.8747, 33) -> (22.5247, 33)
  line L22 (22.5247, 33) -> (22.5247, 39.35)
  line L23 (22.5247, 39.35) -> (28.8747, 39.35)
  line L24 (28.8747, -36.3826) -> (22.5247, -36.3826)
  line L25 (22.5247, -36.3826) -> (22.5247, -30.0326)
  line L26 (22.5247, -30.0326) -> (28.8747, -30.0326)
  line L27 (28.8747, -30.0326) -> (28.8747, -36.3826)
  line L28 (0.425, -77.22) -> (0.425, -82.3)
  line L29 (0.425, -82.3) -> (-5.925, -82.3)
  line L30 (-5.925, -82.3) -> (-5.925, -77.22)
  line L31 (-5.925, -77.22) -> (0.425, -77.22)
  line L32 (0.425, -89.92) -> (0.425, -95)
  line L33 (0.425, -95) -> (-5.925, -95)
  line L34 (-5.925, -95) -> (-5.925, -89.92)
  line L35 (-5.925, -89.92) -> (0.425, -89.92)
  line L36 (16.825, -63) -> (-22.325, -63)
  line L37 (-22.325, -63) -> (-22.325, -30)
  line L38 (-22.325, -30) -> (-25.5, -30)
  line L39 (-25.5, -30) -> (-25.5, 33)
  line L40 (-25.5, 33) -> (-22.325, 33)
  line L41 (-22.325, 33) -> (-22.325, -30)
  line L42 (-22.325, -30) -> (-22.325, -30)
  line L43 (-22.325, -30) -> (-22.325, 66.1383)
  line L44 (-22.325, 66.1383) -> (16.825, 66.1383)
  line L45 (16.825, 66.1383) -> (16.825, 33)
  line L46 (16.825, 33) -> (20, 33)
  line L47 (20, 33) -> (20, -30)
  line L48 (20, -30) -> (16.825, -30)
  line L49 (16.825, -30) -> (16.825, -63)
  line L50 (-123.925, -63) -> (-22.325, -101.1)
  line L51 (-22.325, -101.1) -> (16.825, -101.1)
  line L52 (16.825, -101.1) -> (136.8247, -62.7138)
  line L53 (136.8247, -62.7138) -> (136.8247, 66.4242)
  line L54 (136.8247, 66.4242) -> (16.825, 104.2383)
  line L55 (16.825, 104.2383) -> (-22.325, 104.2383)
  line L56 (-22.325, 104.2383) -> (-123.925, 66.1383)
  line L57 (-123.925, 66.1383) -> (-123.925, -63)
  line L58 (-12.975, -94.75) -> (-19.325, -94.75)
  line L59 (-19.325, -94.75) -> (-19.325, -88.4)
  line L60 (-19.325, -88.4) -> (-12.975, -88.4)
  line L61 (-12.975, -88.4) -> (-12.975, -94.75)
  line L62 (13.825, -94.74) -> (7.475, -94.74)
  line L63 (7.475, -94.74) -> (7.475, -88.39)
  line L64 (7.475, -88.39) -> (13.825, -88.39)
  line L65 (13.825, -88.39) -> (13.825, -94.74)
  line L66 (13.825, 97.8883) -> (7.475, 97.8883)
  line L67 (7.475, 97.8883) -> (7.475, 91.5383)
  line L68 (7.475, 91.5383) -> (13.825, 91.5383)
  line L69 (13.825, 91.5383) -> (13.825, 97.8883)
  line L70 (-12.975, 97.8883) -> (-19.325, 97.8883)
  line L71 (-19.325, 97.8883) -> (-19.325, 91.5383)
  line L72 (-19.325, 91.5383) -> (-12.975, 91.5383)
  line L73 (-12.975, 91.5383) -> (-12.975, 97.8883)
  line L74 (130.4747, -52.7138) -> (124.1247, -52.7138)
  line L75 (124.1247, -52.7138) -> (124.1247, -46.3638)
  line L76 (124.1247, -46.3638) -> (130.4747, -46.3638)
  line L77 (130.4747, -46.3638) -> (130.4747, -52.7138)
  line L78 (130.4747, 50.0742) -> (124.1247, 50.0742)
  line L79 (124.1247, 50.0742) -> (124.1247, 56.4242)
  line L80 (124.1247, 56.4242) -> (130.4747, 56.4242)
  line L81 (130.4747, 56.4242) -> (130.4747, 50.0742)
  line L82 (-117.575, 56.1383) -> (-111.225, 56.1383)
  line L83 (-111.225, 56.1383) -> (-111.225, 49.7883)
  line L84 (-111.225, 49.7883) -> (-117.575, 49.7883)
  line L85 (-117.575, 49.7883) -> (-117.575, 56.1383)
  line L86 (-111.225, -53) -> (-117.575, -53)
  line L87 (-117.575, -53) -> (-117.575, -46.65)
  line L88 (-117.575, -46.65) -> (-111.225, -46.65)
  line L89 (-111.225, -46.65) -> (-111.225, -53)
  dimension "d169" = 6.35
  dimension "d170" = 6.35
  dimension "d171" = 3
  dimension "d172" = 6.35
  dimension "d173" = 6.35
  dimension "d174" = 3
  dimension "d175" = 6.36
  dimension "d176" = 6.35
  dimension "d177" = 20.45
  dimension "d178" = 6.35
  dimension "d179" = 6.35
  dimension "d180" = 6.35
  dimension "d181" = 6.35
  dimension "d182" = 3
  dimension "d184" = 3
  dimension "d185" = 6.35
  dimension "d186" = 6.35
  dimension "d187" = 20.45
  dimension "d188" = 6.35
  dimension "d189" = 6.35
  dimension "d190" = 6.35
  dimension "d191" = 10
  dimension "d192" = 6.35
  dimension "d193" = 6.35
  dimension "d194" = 10
  dimension "d195" = 6.35
  dimension "d196" = 6.35
  dimension "d197" = 6.35
  dimension "d198" = 10
  dimension "d199" = 6.35
  dimension "d200" = 6.35
  dimension "d201" = 6.35
  dimension "d202" = 10
  dimension "d203" = 6.35
  constraint horizontal L58
  constraint vertical L59
  constraint horizontal L60
  constraint vertical L61
  constraint horizontal L62
  constraint vertical L63
  constraint horizontal L64
  constraint vertical L65
  constraint horizontal L66
  constraint vertical L67
  constraint horizontal L68
  constraint vertical L69
  constraint horizontal L70
  constraint vertical L71
  constraint horizontal L72
  constraint vertical L73
  constraint horizontal L74
  constraint vertical L75
  constraint horizontal L76
  constraint vertical L77
  constraint horizontal L78
  constraint vertical L79
  constraint horizontal L80
  constraint vertical L81
  constraint horizontal L82
  constraint vertical L83
  constraint horizontal L84
  constraint vertical L85
  constraint horizontal L86
  constraint vertical L87
  constraint horizontal L88
  constraint vertical L89
  measures "d169" distance of L58.start L58.end
  measures "d170" distance of L58.start L60.end
  measures "d171" distance of L50.end L59
  measures "d172" distance of L62.end L63.end
  measures "d173" distance of L62.start L62.end
  measures "d174" distance of L51.end L65
  measures "d175" distance of L51 L62
  measures "d176" distance of L51 L58
  measures "d177" distance of L61 L63
  measures "d178" distance of L66.start L66.end
  measures "d179" distance of L66.start L68.end
  measures "d180" distance of L70.start L70.end
  measures "d181" distance of L70.start L72.end
  measures "d182" distance of L55.end L71
  measures "d184" distance of L54.end L69
  measures "d185" distance of L55 L66
  measures "d186" distance of L55 L70
  measures "d187" distance of L67 L73
  measures "d188" distance of L74.start L74.end
  measures "d189" distance of L74.end L75.end
  measures "d190" distance of L53 L77
  measures "d191" distance of L52.end L74
  measures "d192" distance of L78.start L80.end
  measures "d193" distance of L78.start L78.end
  measures "d194" distance of L53.end L80
  measures "d195" distance of L53 L81
  measures "d196" distance of L82.start L82.end
  measures "d197" distance of L82.start L84.end
  measures "d198" distance of L56.end L82
  measures "d199" distance of L57 L85
  measures "d200" distance of L86.start L86.end
  measures "d201" distance of L86.start L88.end
  measures "d202" distance of L50.start L86
  measures "d203" distance of L57 L87
extrude "Extrude18" cut sketch "Sketch18" against normal blind 100 contours L58 L59 L60 L61 | L62 L63 L64 L65 | L66 L67 L68 L69 | L70 L71 L72 L73 | L74 L75 L76 L77 | L78 L79 L80 L81 | L82 L83 L84 L85 | L86 L87 L88 L89 bodies 1
